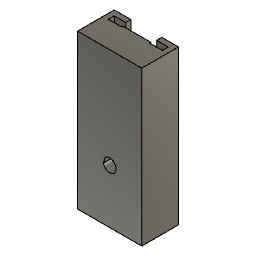
_track for mic.b1789ba0-cf51-4915-8dbb-693580e8ea0b (Autodesk Fusion 360 design; units mm, degrees)
Autodesk Fusion 360 part; units mm, degrees
sketch "Sketch1" plane through (0, 0, 0) normal (0, 0, 1) x (1, 0, 0)
  line L0 (12.5, -5) -> (-12.5, -5)
  line L1 (-12.5, -5) -> (-12.5, 5)
  line L2 (12.5, 5) -> (12.5, -5)
  line L3 (12.5, -5) -> (-12.5, 5) construction
  line L4 (-12.5, -5) -> (12.5, 5) construction
  line L5 (12.5, 5) -> (12.5, 7.3)
  line L6 (10.5, 7.3) -> (10.5, 5)
  line L7 (-5.5, 5.5) -> (5.5, 5.5)
  line L8 (5.5, 5.5) -> (5.5, 5)
  line L9 (-5.5, 5) -> (-5.5, 5.5)
  line L10 (6, 9.3) -> (12.5, 9.3)
  line L11 (12.5, 9.3) -> (12.5, 7.3)
  line L12 (10.5, 7.3) -> (6, 7.3)
  line L13 (6, 7.3) -> (6, 9.3)
  line L14 (-10.5, 5) -> (-5.5, 5)
  line L15 (5.5, 5) -> (10.5, 5)
  line L16 (0, 5.5) -> (0, -5) construction
  line L17 (-6, 7.3) -> (-6, 9.3)
  line L18 (-12.5, 9.3) -> (-12.5, 7.3)
  line L19 (-10.5, 7.3) -> (-10.5, 5)
  line L20 (-12.5, 5) -> (-12.5, 7.3)
  line L21 (-10.5, 7.3) -> (-6, 7.3)
  line L22 (-6, 9.3) -> (-12.5, 9.3)
  dimension "d3" = 25
  dimension "d5" = 10
  dimension "d11" = 11
  dimension "d13" = 0.5
  dimension "d14" = 2.3
  dimension "d17" = 6.5
  dimension "d18" = 2
  constraint horizontal L0
  constraint perpendicular L0 L1
  constraint parallel L1 L2
  constraint coincident L3 origin
  constraint coincident L4 origin
  constraint vertical L5
  constraint perpendicular L2 L14
  constraint perpendicular L6 L14
  constraint horizontal L7
  constraint vertical L8
  constraint vertical L9
  constraint horizontal L10
  constraint vertical L11
  constraint horizontal L12
  constraint vertical L13
  constraint coincident L5.end L11.end
  constraint collinear L14 L15
  constraint midpoint L7 L16.start
  constraint midpoint L0 L16.end
  constraint symmetric L2.start L16 L1.end
  constraint symmetric L5.end L16 L18.end
  constraint symmetric L6.start L16 L19.start
  constraint symmetric L6.end L16 L14.start
  constraint symmetric L10.start L16 L17.end
  constraint symmetric L10.end L16 L18.start
  constraint symmetric L12.end L16 L17.start
  measures "d3" distance of L0.start L0.end
  measures "d5" distance of L0.start L2.start
  measures "d11" distance of L7.start L7.end
  measures "d13" distance of L7.end L8.end
  measures "d14" distance of L2.start L5.end
  measures "d17" distance of L10.start L10.end
  measures "d18" distance of L10.end L5.end
extrude "Extrude1" add sketch "Sketch1" along normal blind 30 and the other way blind 30
sketch "Sketch2" plane through (0, -5, 0) normal (0, -1, 0) x (1, 0, 0)
  line L0 (12.5, -30) -> (12.5, 30)
  line L1 (12.5, 30) -> (-12.5, 30)
  line L2 (-12.5, 30) -> (-12.5, -30)
  line L3 (-12.5, -30) -> (12.5, -30)
  circle A0 centre (0, 20) radius 9
  line L4 (0, 30) -> (0, 0) construction
  dimension "d23" = 18
  constraint midpoint L1 L4.start
  constraint coincident L4.end origin
  constraint coincident A0.centre L4
  measures "d23" diameter of A0
extrude "Extrude2" cut sketch "Sketch2" against normal blind 5 contours A0
sketch "Sketch3" plane through (0, -5, 0) normal (0, -1, 0) x (1, 0, 0)
  circle A0 centre (0, 20) radius 9
  line L0 (12.5, -30) -> (12.5, 30)
  line L1 (12.5, 30) -> (-12.5, 30)
  line L2 (-12.5, 30) -> (-12.5, -30)
  line L3 (-12.5, -30) -> (12.5, -30)
  line L4 (0, 11) -> (0, -9) construction
  line L5 (2.3874, -9.7418) -> (8, -9.7418) construction
  line L6 (-2.2435, -8.7604) -> (-1.7674, -7.2318)
  line L7 (-2.2435, -8.7604) -> (-2.4588, -9.4519)
  arc A1 (-2.4588, -9.4519) -> (-1.7674, -7.2318) centre (0, -9) ccw
  point P0 (-9, 20)
  dimension "d26" = 5
  constraint coincident A0 L4.start
  constraint vertical L4
  constraint coincident L4.end A1.centre
  constraint coincident L5.start A1
  constraint horizontal L5
  constraint parallel L6 L7
  measures "d26" diameter of A1
extrude "Extrude3" cut sketch "Sketch3" against normal blind 7 contours L6 L7 A1
extrude "Extrude4" add 1 faces at (1.8705, 0, 22.3455) along direction (0, -1, 0) blind 5
